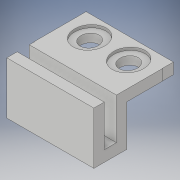
# Autodesk Inventor part: Pantalla - encaix slider
Saved by Autodesk Inventor 2019 (Build 230136000, 136)
## iProperties
Created: 2018-09-18
Part Number: Pantalla - encaix slider
Material: Genérico
Document SubType Name: Modeling
Designer: Albert Garangou Culebras
Density: 1 g/cm^3
Appearance: Valor por defecto
Author: Albert Garangou Culebras
Autodesk Inventor part; units mm, degrees
ref_plane "YZ Plane" through (0, 0, 0) normal (1, 0, 0) x (0, 1, 0)
ref_plane "XZ Plane" through (0, 0, 0) normal (0, 1, 0) x (-1, 0, 0)
ref_plane "XY Plane" through (0, 0, 0) normal (0, 0, 1) x (1, 0, 0)
sketch "Boceto1" plane through (0, 0, 0) normal (0, 1, 0) x (-1, 0, 0)
  line L0 (0, 0) -> (3.5, 0)
  line L1 (3.5, 0) -> (5.5, 0)
  line L2 (0, 0) -> (-2, 0)
  line L3 (-2, -5.5) -> (5.5, -5.5)
  line L4 (-2, 0) -> (-5, 0)
  line L5 (-5, -5.5) -> (-2, -5.5)
  line L6 (5.5, 0) -> (8.5, 0)
  line L7 (8.5, -5.5) -> (5.5, -5.5)
  line L8 (8.5, -5.5) -> (9.5, -5.5)
  line L9 (9.5, 0) -> (8.5, 0)
  line L10 (-5, -5.5) -> (-6, -5.5)
  line L11 (-6, 0) -> (-5, 0)
  line L12 (9.5, -5.5) -> (10.5, -5.5)
  line L13 (10.5, -5.5) -> (10.5, 0)
  line L14 (10.5, 0) -> (9.5, 0)
  line L15 (-6, -5.5) -> (-7, -5.5)
  line L16 (-7, -5.5) -> (-7, 0)
  line L17 (-7, 0) -> (-6, 0)
  dimension "d30" = 1
  dimension "d37" = 1
  dimension "d38" = 1
  constraints: 36 end point, 8 horizontal, 4 perpendicular, 1 collinear, 1 point on line
  measures "d30" distance of L5.start L10.end
  measures "d37" distance of L8.end L12.end
  measures "d38" distance of L10.end L15.end
extrude "Extrusión3" add sketch "Boceto1" along normal blind 2
sketch "Boceto4" plane through (-8.5, 0, 0) normal (0, 0, 1) x (1, 0, 0)
  line L0 (15.5, 2) -> (-2, 2) projected
  line L1 (0, 2) -> (13.5, 2)
  line L2 (13.5, 2) -> (13.5, 0)
  line L3 (13.5, 0) -> (0, 0)
  line L4 (0, 0) -> (0, 2)
  point P0 (8.5, 0)
  point P1 (14.5, 2)
  point P2 (-1, 2)
  constraints: 8 end point, 2 parallel, 1 horizontal, 1 perpendicular
extrude "Extrusión4" add sketch "Boceto4" along normal blind 2
sketch "Boceto13" plane through (0, 2, 0) normal (0, 1, 0) x (1, 0, 0)
  line L0 (7, 5.5) -> (-10.5, 5.5) projected
  line L1 (-10.5, 5.5) -> (6.9708, 5.5)
  line L2 (6.9708, 5.5) -> (6.9708, 7.5)
  line L3 (6.9708, 7.5) -> (-10.5, 7.5)
  line L4 (-10.5, 7.5) -> (-10.5, 5.5)
  point P0 (0, 0)
  point P1 (-8.5, 5.5)
  constraints: 8 end point, 2 parallel, 1 horizontal, 1 perpendicular
extrude "Extrusión13" add sketch "Boceto13" against normal blind 2
sketch "Boceto14" plane through (0, 2, 0) normal (0, 1, 0) x (1, 0, 0)
  circle A0 centre (2.1471, 3.7519) radius 1.75
  circle A1 centre (-5.6769, 3.7519) radius 1.75
  line L0 (1.1471, 3.7519) -> (2.1471, 3.7519)
  line L1 (-4.6769, 3.7519) -> (-5.6769, 3.7519)
  point P0 (0, 0)
  dimension "d43" = 3.5
  dimension "d44" = 3.5
  dimension "d45" = 1
  dimension "d46" = 1
  constraints: 4 end point, 2 centre point, 2 horizontal
  measures "d43" diameter of A0
  measures "d44" diameter of A1
  measures "d45" distance of L0.start L0.end
  measures "d46" distance of L1.start L1.end
extrude "Extrusión14" cut sketch "Boceto14" against normal blind 2
sketch "Boceto15" plane through (0, 2, 0) normal (0, 1, 0) x (1, 0, 0)
  circle A0 centre (2.1471, 3.7519) radius 1.75 projected
  circle A1 centre (2.1471, 3.7519) radius 3
  circle A2 centre (-5.6769, 3.7519) radius 1.75 projected
  circle A3 centre (-5.6769, 3.7519) radius 3
  point P0 (0, 0)
  dimension "d49" = 6
  dimension "d50" = 6
  constraints: 2 centre point, 2 coincident
  measures "d49" diameter of A1
  measures "d50" diameter of A3
extrude "Extrusión15" cut sketch "Boceto15" against normal blind 0.5
sketch "Boceto17" plane through (0, 2, 0) normal (0, 1, 0) x (1, 0, 0)
  line L0 (7, 0) -> (5, 0) projected
  line L1 (7, 0) -> (-10.5, 0)
  line L2 (-10.5, 0) -> (-10.5, -2)
  line L3 (-10.5, -2) -> (7, -2)
  line L4 (7, -2) -> (7, 0)
  point P0 (0, 0)
  dimension "d55" = 17.5
  constraints: 8 end point, 2 parallel, 1 horizontal, 1 perpendicular
  measures "d55" distance of L3.end L2.end
extrude "Extrusión17" add sketch "Boceto17" against normal blind 2
sketch "Boceto18" plane through (-8.5, 0, 2) normal (0, 0, 1) x (1, 0, 0)
  line L0 (-2, 2) -> (15.5, 2) projected
  line L1 (-1.9353, 0) -> (15.5, 0)
  line L2 (15.5, 0) -> (15.5, 2)
  line L3 (15.5, 2) -> (-1.9353, 2)
  line L4 (-1.9353, 2) -> (-1.9353, 0)
  point P0 (8.5, 0)
  constraints: 8 end point, 2 parallel, 1 horizontal, 1 perpendicular
extrude "Extrusión18" add sketch "Boceto18" along normal blind 5
sketch "Boceto19" plane through (0, 0, 0) normal (0, -1, 0) x (1, 0, 0)
  line L0 (-10.5, -7.5) -> (-10.5, 2) projected
  line L1 (-10.4353, 2.9) -> (7, 2.9)
  line L2 (7, 2.9) -> (7, 1)
  line L3 (7, 1) -> (-10.5, 1)
  line L4 (-10.4353, 2.9) -> (-10.5, 1)
  line L5 (7, 7) -> (-10.4353, 7) projected
  line L6 (7, 7) -> (7, 5.1)
  line L7 (7, 7) -> (7, -5.5) projected
  line L8 (7, 5.1) -> (-10.4353, 5.1)
  line L9 (-10.4353, 2) -> (-10.4353, 7) projected
  line L10 (-10.4353, 7) -> (-10.4353, 5.1)
  line L11 (-10.4353, 7) -> (7, 7)
  point P0 (7, 1.001)
  dimension "d67" = 1.9
  dimension "d68" = 1.9
  constraints: 16 end point, 3 perpendicular, 3 point on line, 1 collinear
  measures "d67" distance of L1.end L2.end
  measures "d68" distance of L5.start L6.end
extrude "Extrusión20" add sketch "Boceto19" along normal blind 7.5 contours L1 L2 L3 L4 | L9 L5 L6 L8
sketch "Boceto21" plane through (-10.4353, 0, 2.9) normal (0, 0, 1) x (1, 0, 0)
  line L0 (17.4353, 0) -> (17.4353, -7.5) projected
  line L1 (0, 2) -> (0, -7.5) projected
  line L2 (17.4353, -7.5) -> (0, -7.5)
  line L3 (0, -7.5) -> (0, -5.5)
  line L4 (0, -5.5) -> (17.4353, -5.5)
  line L5 (17.4353, -5.5) -> (17.4353, -7.5)
  point P0 (10.4353, 0)
  dimension "d71" = 2
  constraints: 8 end point, 2 parallel, 1 horizontal, 1 perpendicular, 1 point on line
  measures "d71" distance of L2.end L3.end
extrude "Extrusión21" add sketch "Boceto21" along normal blind 4
sketch "Boceto22" plane through (0, 0, 0) normal (0, -1, 0) x (1, 0, 0)
  line L0 (-10.4353, 2.9) -> (-10.4353, 5.1) projected
  line L1 (7, 2.9) -> (-10.4353, 2.9)
  line L2 (-10.4353, 2.9) -> (-10.4353, 5.1)
  line L3 (-10.4353, 5.1) -> (7, 5.1)
  line L4 (7, 5.1) -> (7, 2.9)
  point P0 (0, 0)
  constraints: 8 end point, 2 parallel, 1 horizontal, 1 perpendicular
extrude "Extrusión22" cut sketch "Boceto22" against normal blind 6.25
scale "Escala1" factors (1, 1, 1.1) then translate (0, 0, -0.7) bodies 1
scale "Escala2" factors (1, 1.1, 1) then translate (0, 0.275, 0) bodies 1
